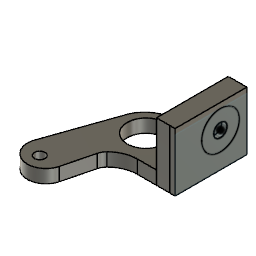
ACOPLE_RUEDA_BARRA_IZQ (Autodesk Fusion 360 design; units mm, degrees)
Autodesk Fusion 360 part; units mm, degrees
sketch "Boceto2" plane through (0, 0, 0) normal (0, 0, 1) x (1, 0, 0)
  circle A0 centre (0, 0) radius 2.5
  circle A1 centre (0, 0) radius 7
  circle A2 centre (12.6785, -27.1892) radius 2
  line L0 (0, 0) -> (12.6785, -27.1892) construction
  line L1 (12.6785, -27.1892) -> (14, -27.1892) construction
  line L2 (-14, 10) -> (-1.0383, 10)
  line L3 (-6.8217, -10) -> (-14, -10)
  line L4 (18.8818, -23.7213) -> (9.5071, 3.1073)
  line L5 (-14, -10) -> (-14, 17)
  arc A3 (1.2721, -13.3803) -> (-6.8217, -10) centre (-6.8217, -21.38) ccw
  line L6 (2.5649, -15.6756) -> (5.4387, -27.1021)
  arc A4 (2.5649, -15.6756) -> (1.2721, -13.3803) centre (-2.2841, -16.8951) ccw
  line L7 (-14, 17) -> (-21, 17)
  line L8 (-21, 17) -> (-21, -10)
  line L9 (-21, -10) -> (-14, -10)
  arc A5 (9.5071, 3.1073) -> (-1.0383, 10) centre (-1.0383, -1.5134) ccw
  line L10 (5.4387, -27.1021) -> (18.8818, -23.7213) construction
  arc A6 (5.4387, -27.1021) -> (18.8818, -23.7213) centre (12.1602, -25.4117) ccw
  line L11 (-21, -35) -> (-21, 19.9655) construction
  circle A7 centre (-42, 0) radius 2.5
  line L12 (-54.6785, -27.1892) -> (-56, -27.1892) construction
  arc A8 (-43.2721, -13.3803) -> (-44.5649, -15.6756) centre (-39.7159, -16.8951) ccw
  line L13 (-35.1783, -10) -> (-28, -10)
  line L14 (-28, -10) -> (-28, 17)
  line L15 (-47.4387, -27.1021) -> (-60.8818, -23.7213) construction
  arc A9 (-35.1783, -10) -> (-43.2721, -13.3803) centre (-35.1783, -21.38) ccw
  line L16 (-21, -10) -> (-28, -10)
  arc A10 (-60.8818, -23.7213) -> (-47.4387, -27.1021) centre (-54.1602, -25.4117) ccw
  circle A11 centre (-42, 0) radius 7
  circle A12 centre (-54.6785, -27.1892) radius 2
  line L17 (-21, 17) -> (-21, -10)
  line L18 (-42, 0) -> (-54.6785, -27.1892) construction
  arc A13 (-40.9617, 10) -> (-51.5071, 3.1073) centre (-40.9617, -1.5134) ccw
  line L19 (-44.5649, -15.6756) -> (-47.4387, -27.1021)
  line L20 (-60.8818, -23.7213) -> (-51.5071, 3.1073)
  line L21 (-28, 10) -> (-40.9617, 10)
  line L22 (-28, 17) -> (-21, 17)
  point P0 (-21, -35)
  point P1 (-21, 19.9655)
  point P2 (-42, 0)
  dimension "d11" = 5
  dimension "d12" = 14
  dimension "d13" = 4
  dimension "d14" = 30
  dimension "d15" = 65
  dimension "d16" = 10
  dimension "d18" = 10
  dimension "d19" = 7
  dimension "d23" = 14
  dimension "d24" = 5
  dimension "d26" = 7
  dimension "d27" = 10
  dimension "d29" = 7
  dimension "d30" = 27
  constraint coincident A0.centre A1.centre
  constraint concentric A0 A1
  constraint coincident A2.centre L0.end
  constraint horizontal L1
  constraint horizontal L2
  constraint horizontal L3
  constraint vertical L5
  constraint coincident L2.start L5
  constraint tangent L3 A3
  constraint tangent A3 A4
  constraint tangent L6 A4
  constraint perpendicular L5 L7
  constraint perpendicular L7 L8
  constraint tangent L2 A5
  constraint perpendicular L6 L10
  constraint tangent L6 A6
  constraint perpendicular L7 L11
  constraint symmetric A0.centre L11 P2
  constraint symmetric A0 L11 A7
  constraint symmetric A1 L11 A11
  constraint symmetric A2 L11 A12
  constraint symmetric A2.centre L11 L12.start
  constraint symmetric L1.end L11 L12.end
  constraint symmetric L2.start L11 L21.start
  constraint symmetric L3.end L11 L13.end
  constraint symmetric L2.end L11 A13.start
  constraint symmetric L4.end L11 A13.end
  constraint symmetric L3.start L11 L13.start
  constraint symmetric L5.end L11 L14.end
  constraint symmetric A3 L11 A9
  constraint symmetric L6.start L11 A8.end
  constraint symmetric A3.start L11 A8.start
  constraint symmetric A4 L11 A8
  constraint symmetric L7.end L11 L8.start
  constraint symmetric L8.end L11 L9.start
  constraint symmetric A5 L11 A13
  constraint symmetric L6.end L11 L15.start
  constraint symmetric L4.start L11 L15.end
  constraint symmetric A6 L11 A10
  constraint symmetric P0 L11 L11.start
  constraint symmetric P1 L11 L11.end
  measures "d11" diameter of A0
  measures "d12" diameter of A1
  measures "d13" diameter of A2
  measures "d14" distance of A0.centre A2.centre
  measures "d15" angle of L0 L1
  measures "d16" distance of A0.centre L2
  measures "d18" distance of A0.centre L4
  measures "d19" distance of A2.centre L4
  measures "d23" distance of A0.centre L5
  measures "d24" radius of A4
  measures "d26" distance of A2.centre L6
  measures "d27" distance of A0.centre L3
  measures "d29" distance of L5 L8
  measures "d30" distance of L7 L9
sketch "Boceto3" plane through (-21, 0, 0) normal (-1, 0, 0) x (0, -1, 0)
  line L0 (-17, 0) -> (10, 0)
  line L1 (10, 0) -> (10, 20)
  line L2 (10, 20) -> (-17, 20)
  line L3 (-17, 20) -> (-17, 0)
  circle A0 centre (-7, 13) radius 7.05
  circle A1 centre (-7, 13) radius 2.5
  dimension "d38" = 14.1
  dimension "d39" = 10
  dimension "d40" = 7
  dimension "d41" = 5
  constraint concentric A0 A1
  measures "d38" diameter of A0
  measures "d39" distance of L3 A0.centre
  measures "d40" distance of L2 A0.centre
  measures "d41" diameter of A1
extrude "Extruir8" add sketch "Boceto2" along normal blind 5 contours A8 L13 L14 A9 A10 A13 L19 L20 L21
extrude "Extruir9" add sketch "Boceto2" along normal blind 5 contours A11
extrude "Extruir10" add sketch "Boceto2" along normal blind 22 contours L8 L14 L16 L17 L22
extrude "Extruir11" cut sketch "Boceto3" along normal blind 8 contours A1
extrude "Extruir12" cut sketch "Boceto3" along normal blind 14 contours L2 A0 | L2 A0
fillet "Empalme1" radius 2 1 edges at (-28, 10, 2.5)
extrude "Extruir13" cut sketch "Boceto2" along normal blind 15 contours A11
move_face "CarasDesfase1" offset -2 1 faces at (-21, -6.6571, 11.3164)
extrude "Extruir14" add 1 faces at (-23, -6.6571, 11.3164) along direction (1, 0, 0) blind 2
extrude "Extruir15" add sketch "Boceto3" along normal blind 2 contours L2 A0 | L2 A0
